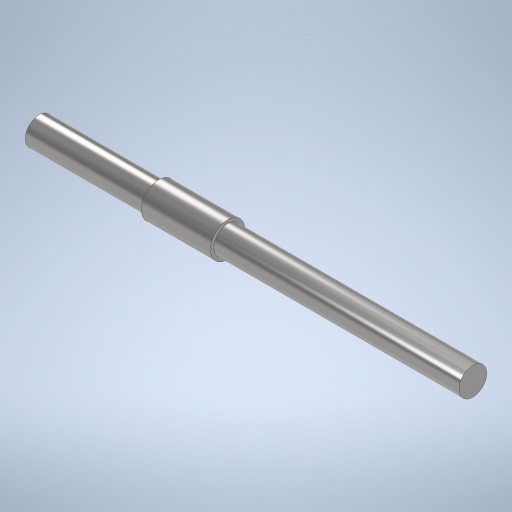
# Autodesk Inventor part: shoulder2_shaft
Saved by Autodesk Inventor 2024 (Build 280153000, 153)
## iProperties
Created: 2025-08-07
Part Number: shoulder2_shaft
Material: 鋼、炭素鋼
Document SubType Name: Modeling
Designer: HosodaLab2
Density: 7.85 g/cm^3
Appearance: 半つや出し
個数: 1
Author: HosodaLab2
Autodesk Inventor part; units mm, degrees
ref_plane "YZ Plane" through (0, 0, 0) normal (1, 0, 0) x (0, 1, 0)
sketch "スケッチ1" plane through (0, 0, 0) normal (0, 1, 0) x (-1, 0, 0)
  circle A0 centre (0, 0) radius 5
  dimension "d0" = 10
  constraints: 1 centre point, 1 coincident
  measures "d0" diameter of A0
extrude "押し出し1" add sketch "スケッチ1" along normal blind 20
sketch "スケッチ2" plane through (0, 20, 0) normal (0, 1, 0) x (1, 0, 0)
  circle A0 centre (0, 0) radius 4
  dimension "d3" = 8
  constraints: 1 centre point, 1 coincident
  measures "d3" diameter of A0
extrude "押し出し2" add sketch "スケッチ2" along normal blind 71
sketch "スケッチ3" plane through (0, 0, 0) normal (0, -1, 0) x (1, 0, 0)
  circle A0 centre (0, 0) radius 4
  dimension "d6" = 8
  constraints: 1 centre point, 1 coincident
  measures "d6" diameter of A0
extrude "押し出し3" add sketch "スケッチ3" along normal blind 34.6
sketch "スケッチ4" plane through (0, -34.6, 0) normal (0, -1, 0) x (1, 0, 0)
  circle A0 centre (0, 0) radius 4 projected
  point P0 (0, 4)
  constraints: 1 vertical alignment, 1 other
ref_plane "作業平面1" through (0, -34.6, 4) normal (0, 0, 1) x (1, 0, 0)
sketch "スケッチ7" plane through (0, -34.6, 4) normal (0, 0, 1) x (1, 0, 0)
  line L0 (-1.5, 5) -> (1.5, 5)
  line L1 (1.5, 5) -> (1.5, 21)
  line L2 (1.5, 21) -> (-1.5, 21)
  line L3 (-1.5, 21) -> (-1.5, 5)
  line L4 (-1.5, 5) -> (1.5, 21) construction
  line L5 (1.5, 5) -> (-1.5, 21) construction
  line L6 (-4, 0) -> (4, 0) projected
  line L7 (-1.5, 104.6) -> (1.5, 104.6)
  line L8 (1.5, 104.6) -> (1.5, 120.6)
  line L9 (1.5, 120.6) -> (-1.5, 120.6)
  line L10 (-1.5, 120.6) -> (-1.5, 104.6)
  line L11 (-1.5, 104.6) -> (1.5, 120.6) construction
  line L12 (1.5, 104.6) -> (-1.5, 120.6) construction
  line L13 (4, 125.6) -> (-4, 125.6) projected
  point P0 (0, 34.6)
  point P1 (0, 13)
  point P2 (0, 112.6)
  dimension "d17" = 3
  dimension "d18" = 16
  dimension "d19" = 5
  dimension "d20" = 3
  dimension "d21" = 16
  dimension "d22" = 5
  constraints: 24 end point, 4 midpoint, 4 parallel, 2 horizontal, 2 perpendicular
  measures "d17" distance of L2.end L1.end
  measures "d18" distance of L1.end L0.end
  measures "d19" distance between parallel lines of L6 L0
  measures "d20" distance of L9.end L8.end
  measures "d21" distance of L8.end L7.end
  measures "d22" distance between parallel lines of L13 L9
extrude "押し出し5" [suppressed]
sketch "スケッチ8" plane through (0, 20, 0) normal (0, 1, 0) x (1, 0, 0)
  circle A0 centre (0, 0) radius 5
  dimension "d25" = 10
  constraints: 1 centre point, 1 coincident
  measures "d25" diameter of A0
extrude "押し出し6" [suppressed]
sketch "スケッチ9" plane through (0, 0, 0) normal (0, -1, 0) x (1, 0, 0)
  circle A0 centre (0, 0) radius 5 projected
  circle A1 centre (0, 0) radius 5
  dimension "d28" = 10
  constraints: 1 centre point, 1 coincident
  measures "d28" diameter of A1
extrude "押し出し7" [suppressed]
sketch "スケッチ10" plane through (0, 0, 0) normal (0, -1, 0) x (1, 0, 0)
  circle A0 centre (0, 0) radius 4 projected
  point P0 (-4, 0)
  constraints: 1 horizontal alignment, 1 other
ref_plane "作業平面2" through (-4, 0, 0) normal (-1, 0, 0) x (0, -1, 0)
sketch "スケッチ11" plane through (-4, 0, 0) normal (-1, 0, 0) x (0, -1, 0)
  line L0 (0, -1.5) -> (5, -1.5)
  line L1 (5, -1.5) -> (5, 1.5)
  line L2 (5, 1.5) -> (0, 1.5)
  line L3 (0, 1.5) -> (0, -1.5)
  line L4 (0, -1.5) -> (5, 1.5) construction
  line L5 (5, -1.5) -> (0, 1.5) construction
  line L6 (0, 5) -> (0, -5) projected
  line L7 (-25, 1.5) -> (-20, 1.5)
  line L8 (-20, 1.5) -> (-20, -1.5)
  line L9 (-20, -1.5) -> (-25, -1.5)
  line L10 (-25, -1.5) -> (-25, 1.5)
  line L11 (-25, 1.5) -> (-20, -1.5) construction
  line L12 (-20, 1.5) -> (-25, -1.5) construction
  line L13 (-20, 5) -> (-20, -5) projected
  line L14 (-80, 1.5) -> (-64, 1.5)
  line L15 (-64, 1.5) -> (-64, -1.5)
  line L16 (-64, -1.5) -> (-80, -1.5)
  line L17 (-80, -1.5) -> (-80, 1.5)
  line L18 (-80, 1.5) -> (-64, -1.5) construction
  line L19 (-64, 1.5) -> (-80, -1.5) construction
  line L20 (-91, 4) -> (-91, -4) projected
  point P0 (0, 0)
  point P1 (2.5, 0)
  point P2 (-22.5, 0)
  point P3 (-72, 0)
  dimension "d31" = 5
  dimension "d32" = 3
  dimension "d33" = 0
  dimension "d34" = 5
  dimension "d35" = 3
  dimension "d36" = 0
  dimension "d39" = 16
  dimension "d40" = 3
  dimension "d41" = 11
  constraints: 36 end point, 6 midpoint, 6 parallel, 3 horizontal, 3 perpendicular
  measures "d31" distance of L2.end L1.end
  measures "d32" distance of L1.end L0.end
  measures "d33" distance between parallel lines of L6 L3
  measures "d34" distance of L8.end L9.end
  measures "d35" distance of L7.end L8.end
  measures "d36" distance between parallel lines of L13 L8
  measures "d39" distance of L15.end L16.end
  measures "d40" distance of L14.end L15.end
  measures "d41" distance between parallel lines of L20 L17
extrude "押し出し8" cut sketch "スケッチ11" against normal blind 1.8
